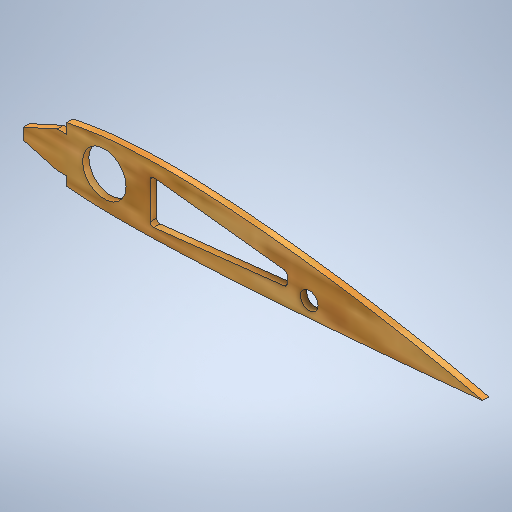
# Autodesk Inventor part: 2414 basic aerofoil
Saved by Autodesk Inventor 2025.1 (Build 291241000, 241)
## iProperties
Created: 2024-11-04
Part Number: 2414 basic aerofoil
Material: Plywood, Finish
Document SubType Name: Modeling
Designer: johan
Density: 0.552 g/cm^3
Appearance: Plywood - New
Author: johan
Autodesk Inventor part; units mm, degrees
ref_plane "YZ Plane" through (0, 0, 0) normal (1, 0, 0) x (0, 1, 0)
ref_plane "XZ Plane" through (0, 0, 0) normal (0, 1, 0) x (-1, 0, 0)
ref_plane "XY Plane" through (0, 0, 0) normal (0, 0, 1) x (1, 0, 0)
sketch "Sketch2" plane through (0, 0, 0) normal (0, 0, 1) x (1, 0, 0)
  spline S0 degree 5 poles (319.6498, 0.0573) (319.6501, 0.0612) (319.6024, 0.0717) (319.3745, 0.1032) (319.3587, 0.1577) (318.7204, 0.2502) (318.4411, 0.3675) (317.6227, 0.5236) (316.9347, 0.7102) (315.9239, 0.9334) (314.8763, 1.1861) (313.6258, 1.4728) (312.2675, 1.7887) (310.7514, 2.1347) (309.1071, 2.5099) (307.3204, 2.9131) (305.4017, 3.3421) (303.3481, 3.7974) (301.1639, 4.2757) (298.8502, 4.7782) (296.4092, 5.301) (293.8432, 5.8446) (291.1548, 6.4061) (288.3466, 6.9857) (285.4207, 7.5803) (282.3807, 8.1894) (279.2284, 8.8107) (275.968, 9.4437) (272.6016, 10.0865) (269.1329, 10.7361) (265.5656, 11.3942) (261.9019, 12.0551) (258.1469, 12.7207) (254.3029, 13.3883) (250.3742, 14.0555) (246.3647, 14.7217) (242.2776, 15.3854) (238.118, 16.0441) (233.8887, 16.6979) (229.5952, 17.3434) (225.2402, 17.981) (220.8297, 18.6074) (216.3658, 19.2226) (211.8552, 19.8242) (207.3009, 20.4107) (202.7077, 20.9813) (198.0804, 21.5339) (193.4232, 22.0679) (188.7413, 22.58) (184.0389, 23.0713) (179.321, 23.5382) (174.592, 23.982) (169.8567, 24.3971) (165.1201, 24.7874) (160.3872, 25.1472) (155.6604, 25.4776) (150.948, 25.7772) (146.2454, 26.0449) (141.5744, 26.278) (136.9015, 26.4795) (132.2479, 26.6311) (127.6319, 26.7393) (123.054, 26.7999) (118.5202, 26.8147) (114.0397, 26.7815) (109.6094, 26.7031) (105.2517, 26.5723) (100.9331, 26.4088) (96.7495, 26.1663) (92.5147, 25.9483) (88.6376, 25.5343) (84.2302, 25.3974) (76.5297, 24.5259) (73.18, 23.8676) (69.3619, 23.413) (65.9721, 22.8018) (62.3454, 22.244) (59.4319, 21.514) (55.4307, 21.0148) (53.2464, 20.1084) (49.5889, 19.537) (47.2944, 18.6473) (44.3884, 17.909) (41.914, 17.071) (39.4431, 16.2394) (37.1538, 15.3738) (34.9769, 14.4941) (32.9455, 13.5944) (31.0501, 12.6807) (29.2961, 11.7542) (27.6837, 10.8151) (26.2149, 9.8673) (24.8895, 8.9103) (23.7099, 7.9467) (22.6751, 6.976) (21.7868, 6.0004) (21.0458, 5.0186) (20.4526, 4.032) (20.0117, 3.0392) (19.7221, 2.0438) (19.5893, 1.0479) (19.6118, 0.0538) (19.7865, -0.9258) (20.1138, -1.8742) (20.591, -2.7944) (21.2165, -3.6796) (21.9855, -4.5321) (22.8956, -5.3514) (23.9453, -6.1385) (25.1332, -6.8944) (26.4582, -7.6188) (27.9184, -8.3123) (29.5136, -8.9751) (31.2409, -9.6071) (33.0997, -10.2067) (35.0892, -10.7758) (37.2002, -11.3131) (39.4562, -11.8174) (41.7927, -12.2939) (44.3651, -12.7275) (46.7744, -13.1584) (50.0005, -13.481) (52.1533, -13.8927) (55.9371, -14.1294) (58.2153, -14.4717) (61.732, -14.6854) (64.8012, -14.9153) (68.2287, -15.092) (71.6338, -15.2498) (75.1915, -15.3722) (78.8138, -15.4692) (82.5326, -15.5359) (86.3291, -15.5764) (90.2061, -15.5901) (94.1575, -15.5787) (98.1812, -15.5438) (102.2727, -15.4851) (106.4286, -15.4059) (110.6456, -15.3062) (114.9188, -15.1867) (119.2459, -15.0512) (123.6218, -14.8988) (128.0442, -14.7319) (132.5111, -14.552) (137.0141, -14.3592) (141.5621, -14.1606) (146.1675, -13.9403) (150.787, -13.7052) (155.434, -13.4523) (160.0951, -13.1857) (164.7676, -12.9046) (169.4465, -12.6129) (174.1261, -12.3082) (178.8033, -11.9955) (183.4722, -11.6727) (188.1294, -11.3426) (192.7696, -11.0072) (197.3886, -10.6641) (201.9818, -10.3188) (206.5448, -9.9678) (211.0728, -9.6157) (215.5623, -9.2611) (220.0069, -8.9047) (224.4048, -8.5497) (228.7492, -8.193) (233.0373, -7.8393) (237.2647, -7.4865) (241.4259, -7.1353) (245.5189, -6.7884) (249.5374, -6.4441) (253.4791, -6.104) (257.3389, -5.7683) (261.1136, -5.4376) (264.7987, -5.113) (268.3914, -4.7937) (271.8871, -4.4807) (275.2826, -4.1749) (278.5752, -3.8759) (281.7596, -3.585) (284.8354, -3.3021) (287.7962, -3.0278) (290.6419, -2.763) (293.3672, -2.5063) (295.9712, -2.2616) (298.4496, -2.0246) (300.8012, -1.801) (303.0222, -1.5859) (305.1122, -1.3849) (307.0656, -1.194) (308.8864, -1.0166) (310.5623, -0.8504) (312.1091, -0.6993) (313.4945, -0.5587) (314.7717, -0.4371) (315.8415, -0.3205) (316.8737, -0.2329) (317.5782, -0.1363) (318.4119, -0.0906) (318.7016, -0.0103) (319.3493, -0.0034) (319.3699, 0.0485) (319.6005, 0.0494) (319.6495, 0.0534) (319.6498, 0.0573) knots 0 0 0 0 0 0 1 2 3 4 5 6 7 8 9 10 11 12 13 14 15 16 17 18 19 20 21 22 23 24 25 26 27 28 29 30 31 32 33 34 35 36 37 38 39 40 41 42 43 44 45 46 47 48 49 50 51 52 53 54 55 56 57 58 59 60 61 62 63 64 65 66 67 68 69 70 71 72 73 74 75 76 77 78 79 80 81 82 83 84 85 86 87 88 89 90 91 92 93 94 95 96 97 98 99 100 101 102 103 104 105 106 107 108 109 110 111 112 113 114 115 116 117 118 119 120 121 122 123 124 125 126 127 128 129 130 131 132 133 134 135 136 137 138 139 140 141 142 143 144 145 146 147 148 149 150 151 152 153 154 155 156 157 158 159 160 161 162 163 164 165 166 167 168 169 170 171 172 173 174 175 176 177 178 179 180 181 182 183 184 185 186 187 188 189 190 191 192 193 194 195 196 197 198 199 199 199 199 199 199
  circle A0 centre (79.5137, 4.5678) radius 13.838
  line L0 (79.5137, 4.5678) -> (79.5137, -15.4763) construction
  line L1 (79.5137, 4.5678) -> (209.6498, 4.5678) construction
  line L2 (319.6498, 0.0573) -> (219.6498, 0.0573) construction
  line L3 (319.6498, 0.0573) -> (319.6498, 0.0574) construction
  line L4 (28.0058, 4.5054) -> (28.0058, -2.4946)
  line L5 (19.6272, 1.0326) -> (319.6498, 0.0573) construction
  line L6 (49.7105, 14.4213) -> (55.6078, 14.4213)
  line L7 (49.7104, -8.4914) -> (55.6078, -8.4914)
  line L8 (28.0058, 4.5054) -> (49.7105, 14.4213)
  line L9 (28.0058, -2.4946) -> (49.7104, -8.4914)
  line L10 (55.6078, 14.4213) -> (55.6078, 20.8729)
  line L11 (55.6078, -8.4914) -> (55.6078, -14.1513)
  line L12 (108.6496, 16.3299) -> (108.6496, -7.1942)
  line L13 (110.8735, -9.1817) -> (193.8736, 0.1678)
  line L14 (195.6498, 2.1552) -> (195.6498, 6.9805)
  line L15 (193.8736, 8.9679) -> (110.8735, 18.3173)
  arc A1 (110.8735, 18.3173) -> (108.6496, 16.3299) centre (110.6496, 16.3299) ccw
  arc A2 (108.6496, -7.1942) -> (110.8735, -9.1817) centre (110.6496, -7.1942) ccw
  arc A3 (193.8736, 0.1678) -> (195.6498, 2.1552) centre (193.6498, 2.1552) ccw
  arc A4 (195.6498, 6.9805) -> (193.8736, 8.9679) centre (193.6498, 6.9805) ccw
  circle A5 centre (209.6498, 0.0573) radius 5.661
  line L16 (319.6498, 0.0573) -> (319.6501, 0.0612) construction
  line L17 (319.6501, 0.0612) -> (319.6024, 0.0717) construction
  line L18 (319.6024, 0.0717) -> (319.3745, 0.1032) construction
  line L19 (319.3745, 0.1032) -> (319.3587, 0.1577) construction
  line L20 (319.3587, 0.1577) -> (318.7204, 0.2502) construction
  line L21 (318.7204, 0.2502) -> (318.4411, 0.3675) construction
  line L22 (318.4411, 0.3675) -> (317.6227, 0.5236) construction
  line L23 (317.6227, 0.5236) -> (316.9347, 0.7102) construction
  line L24 (316.9347, 0.7102) -> (315.9239, 0.9334) construction
  line L25 (315.9239, 0.9334) -> (314.8763, 1.1861) construction
  line L26 (314.8763, 1.1861) -> (313.6258, 1.4728) construction
  line L27 (313.6258, 1.4728) -> (312.2675, 1.7887) construction
  line L28 (312.2675, 1.7887) -> (310.7514, 2.1347) construction
  line L29 (310.7514, 2.1347) -> (309.1071, 2.5099) construction
  line L30 (309.1071, 2.5099) -> (307.3204, 2.9131) construction
  line L31 (307.3204, 2.9131) -> (305.4017, 3.3421) construction
  line L32 (305.4017, 3.3421) -> (303.3481, 3.7974) construction
  line L33 (303.3481, 3.7974) -> (301.1639, 4.2757) construction
  line L34 (301.1639, 4.2757) -> (298.8502, 4.7782) construction
  line L35 (298.8502, 4.7782) -> (296.4092, 5.301) construction
  line L36 (296.4092, 5.301) -> (293.8432, 5.8446) construction
  line L37 (293.8432, 5.8446) -> (291.1548, 6.4061) construction
  line L38 (291.1548, 6.4061) -> (288.3466, 6.9857) construction
  line L39 (288.3466, 6.9857) -> (285.4207, 7.5803) construction
  line L40 (285.4207, 7.5803) -> (282.3807, 8.1894) construction
  line L41 (282.3807, 8.1894) -> (279.2284, 8.8107) construction
  line L42 (279.2284, 8.8107) -> (275.968, 9.4437) construction
  line L43 (275.968, 9.4437) -> (272.6016, 10.0865) construction
  line L44 (272.6016, 10.0865) -> (269.1329, 10.7361) construction
  line L45 (269.1329, 10.7361) -> (265.5656, 11.3942) construction
  line L46 (265.5656, 11.3942) -> (261.9019, 12.0551) construction
  line L47 (261.9019, 12.0551) -> (258.1469, 12.7207) construction
  line L48 (258.1469, 12.7207) -> (254.3029, 13.3883) construction
  line L49 (254.3029, 13.3883) -> (250.3742, 14.0555) construction
  line L50 (250.3742, 14.0555) -> (246.3647, 14.7217) construction
  line L51 (246.3647, 14.7217) -> (242.2776, 15.3854) construction
  line L52 (242.2776, 15.3854) -> (238.118, 16.0441) construction
  line L53 (238.118, 16.0441) -> (233.8887, 16.6979) construction
  line L54 (233.8887, 16.6979) -> (229.5952, 17.3434) construction
  line L55 (229.5952, 17.3434) -> (225.2402, 17.981) construction
  line L56 (225.2402, 17.981) -> (220.8297, 18.6074) construction
  line L57 (220.8297, 18.6074) -> (216.3658, 19.2226) construction
  line L58 (216.3658, 19.2226) -> (211.8552, 19.8242) construction
  line L59 (211.8552, 19.8242) -> (207.3009, 20.4107) construction
  line L60 (207.3009, 20.4107) -> (202.7077, 20.9813) construction
  line L61 (202.7077, 20.9813) -> (198.0804, 21.5339) construction
  line L62 (198.0804, 21.5339) -> (193.4232, 22.0679) construction
  line L63 (193.4232, 22.0679) -> (188.7413, 22.58) construction
  line L64 (188.7413, 22.58) -> (184.0389, 23.0713) construction
  line L65 (184.0389, 23.0713) -> (179.321, 23.5382) construction
  line L66 (179.321, 23.5382) -> (174.592, 23.982) construction
  line L67 (174.592, 23.982) -> (169.8567, 24.3971) construction
  line L68 (169.8567, 24.3971) -> (165.1201, 24.7874) construction
  line L69 (165.1201, 24.7874) -> (160.3872, 25.1472) construction
  line L70 (160.3872, 25.1472) -> (155.6604, 25.4776) construction
  line L71 (155.6604, 25.4776) -> (150.948, 25.7772) construction
  line L72 (150.948, 25.7772) -> (146.2454, 26.0449) construction
  line L73 (146.2454, 26.0449) -> (141.5744, 26.278) construction
  line L74 (141.5744, 26.278) -> (136.9015, 26.4795) construction
  line L75 (136.9015, 26.4795) -> (132.2479, 26.6311) construction
  line L76 (132.2479, 26.6311) -> (127.6319, 26.7393) construction
  line L77 (127.6319, 26.7393) -> (123.054, 26.7999) construction
  line L78 (123.054, 26.7999) -> (118.5202, 26.8147) construction
  line L79 (118.5202, 26.8147) -> (114.0397, 26.7815) construction
  line L80 (114.0397, 26.7815) -> (109.6094, 26.7031) construction
  line L81 (109.6094, 26.7031) -> (105.2517, 26.5723) construction
  line L82 (105.2517, 26.5723) -> (100.9331, 26.4088) construction
  line L83 (100.9331, 26.4088) -> (96.7495, 26.1663) construction
  line L84 (96.7495, 26.1663) -> (92.5147, 25.9483) construction
  line L85 (92.5147, 25.9483) -> (88.6376, 25.5343) construction
  line L86 (88.6376, 25.5343) -> (84.2302, 25.3974) construction
  line L87 (84.2302, 25.3974) -> (76.5297, 24.5259) construction
  line L88 (76.5297, 24.5259) -> (73.18, 23.8676) construction
  line L89 (73.18, 23.8676) -> (69.3619, 23.413) construction
  line L90 (69.3619, 23.413) -> (65.9721, 22.8018) construction
  line L91 (65.9721, 22.8018) -> (62.3454, 22.244) construction
  line L92 (62.3454, 22.244) -> (59.4319, 21.514) construction
  line L93 (59.4319, 21.514) -> (55.4307, 21.0148) construction
  line L94 (55.4307, 21.0148) -> (53.2464, 20.1084) construction
  line L95 (53.2464, 20.1084) -> (49.5889, 19.537) construction
  line L96 (49.5889, 19.537) -> (47.2944, 18.6473) construction
  line L97 (47.2944, 18.6473) -> (44.3884, 17.909) construction
  line L98 (44.3884, 17.909) -> (41.914, 17.071) construction
  line L99 (41.914, 17.071) -> (39.4431, 16.2394) construction
  line L100 (39.4431, 16.2394) -> (37.1538, 15.3738) construction
  line L101 (37.1538, 15.3738) -> (34.9769, 14.4941) construction
  line L102 (34.9769, 14.4941) -> (32.9455, 13.5944) construction
  line L103 (32.9455, 13.5944) -> (31.0501, 12.6807) construction
  line L104 (31.0501, 12.6807) -> (29.2961, 11.7542) construction
  line L105 (29.2961, 11.7542) -> (27.6837, 10.8151) construction
  line L106 (27.6837, 10.8151) -> (26.2149, 9.8673) construction
  line L107 (26.2149, 9.8673) -> (24.8895, 8.9103) construction
  line L108 (24.8895, 8.9103) -> (23.7099, 7.9467) construction
  line L109 (23.7099, 7.9467) -> (22.6751, 6.976) construction
  line L110 (22.6751, 6.976) -> (21.7868, 6.0004) construction
  line L111 (21.7868, 6.0004) -> (21.0458, 5.0186) construction
  line L112 (21.0458, 5.0186) -> (20.4526, 4.032) construction
  line L113 (20.4526, 4.032) -> (20.0117, 3.0392) construction
  line L114 (20.0117, 3.0392) -> (19.7221, 2.0438) construction
  line L115 (19.7221, 2.0438) -> (19.5893, 1.0479) construction
  line L116 (19.5893, 1.0479) -> (19.6118, 0.0538) construction
  line L117 (19.6118, 0.0538) -> (19.7865, -0.9258) construction
  line L118 (19.7865, -0.9258) -> (20.1138, -1.8742) construction
  line L119 (20.1138, -1.8742) -> (20.591, -2.7944) construction
  line L120 (20.591, -2.7944) -> (21.2165, -3.6796) construction
  line L121 (21.2165, -3.6796) -> (21.9855, -4.5321) construction
  line L122 (21.9855, -4.5321) -> (22.8956, -5.3514) construction
  line L123 (22.8956, -5.3514) -> (23.9453, -6.1385) construction
  line L124 (23.9453, -6.1385) -> (25.1332, -6.8944) construction
  line L125 (25.1332, -6.8944) -> (26.4582, -7.6188) construction
  line L126 (26.4582, -7.6188) -> (27.9184, -8.3123) construction
  line L127 (27.9184, -8.3123) -> (29.5136, -8.9751) construction
  line L128 (29.5136, -8.9751) -> (31.2409, -9.6071) construction
  line L129 (31.2409, -9.6071) -> (33.0997, -10.2067) construction
  line L130 (33.0997, -10.2067) -> (35.0892, -10.7758) construction
  line L131 (35.0892, -10.7758) -> (37.2002, -11.3131) construction
  line L132 (37.2002, -11.3131) -> (39.4562, -11.8174) construction
  line L133 (39.4562, -11.8174) -> (41.7927, -12.2939) construction
  line L134 (41.7927, -12.2939) -> (44.3651, -12.7275) construction
  line L135 (44.3651, -12.7275) -> (46.7744, -13.1584) construction
  line L136 (46.7744, -13.1584) -> (50.0005, -13.481) construction
  line L137 (50.0005, -13.481) -> (52.1533, -13.8927) construction
  line L138 (52.1533, -13.8927) -> (55.9371, -14.1294) construction
  line L139 (55.9371, -14.1294) -> (58.2153, -14.4717) construction
  line L140 (58.2153, -14.4717) -> (61.732, -14.6854) construction
  line L141 (61.732, -14.6854) -> (64.8012, -14.9153) construction
  line L142 (64.8012, -14.9153) -> (68.2287, -15.092) construction
  line L143 (68.2287, -15.092) -> (71.6338, -15.2498) construction
  line L144 (71.6338, -15.2498) -> (75.1915, -15.3722) construction
  line L145 (75.1915, -15.3722) -> (78.8138, -15.4692) construction
  line L146 (78.8138, -15.4692) -> (82.5326, -15.5359) construction
  line L147 (82.5326, -15.5359) -> (86.3291, -15.5764) construction
  line L148 (86.3291, -15.5764) -> (90.2061, -15.5901) construction
  line L149 (90.2061, -15.5901) -> (94.1575, -15.5787) construction
  line L150 (94.1575, -15.5787) -> (98.1812, -15.5438) construction
  line L151 (98.1812, -15.5438) -> (102.2727, -15.4851) construction
  line L152 (102.2727, -15.4851) -> (106.4286, -15.4059) construction
  line L153 (106.4286, -15.4059) -> (110.6456, -15.3062) construction
  line L154 (110.6456, -15.3062) -> (114.9188, -15.1867) construction
  line L155 (114.9188, -15.1867) -> (119.2459, -15.0512) construction
  line L156 (119.2459, -15.0512) -> (123.6218, -14.8988) construction
  line L157 (123.6218, -14.8988) -> (128.0442, -14.7319) construction
  line L158 (128.0442, -14.7319) -> (132.5111, -14.552) construction
  line L159 (132.5111, -14.552) -> (137.0141, -14.3592) construction
  line L160 (137.0141, -14.3592) -> (141.5621, -14.1606) construction
  line L161 (141.5621, -14.1606) -> (146.1675, -13.9403) construction
  line L162 (146.1675, -13.9403) -> (150.787, -13.7052) construction
  line L163 (150.787, -13.7052) -> (155.434, -13.4523) construction
  line L164 (155.434, -13.4523) -> (160.0951, -13.1857) construction
  line L165 (160.0951, -13.1857) -> (164.7676, -12.9046) construction
  line L166 (164.7676, -12.9046) -> (169.4465, -12.6129) construction
  line L167 (169.4465, -12.6129) -> (174.1261, -12.3082) construction
  line L168 (174.1261, -12.3082) -> (178.8033, -11.9955) construction
  line L169 (178.8033, -11.9955) -> (183.4722, -11.6727) construction
  line L170 (183.4722, -11.6727) -> (188.1294, -11.3426) construction
  line L171 (188.1294, -11.3426) -> (192.7696, -11.0072) construction
  line L172 (192.7696, -11.0072) -> (197.3886, -10.6641) construction
  line L173 (197.3886, -10.6641) -> (201.9818, -10.3188) construction
  line L174 (201.9818, -10.3188) -> (206.5448, -9.9678) construction
  line L175 (206.5448, -9.9678) -> (211.0728, -9.6157) construction
  line L176 (211.0728, -9.6157) -> (215.5623, -9.2611) construction
  line L177 (215.5623, -9.2611) -> (220.0069, -8.9047) construction
  line L178 (220.0069, -8.9047) -> (224.4048, -8.5497) construction
  line L179 (224.4048, -8.5497) -> (228.7492, -8.193) construction
  line L180 (228.7492, -8.193) -> (233.0373, -7.8393) construction
  line L181 (233.0373, -7.8393) -> (237.2647, -7.4865) construction
  line L182 (237.2647, -7.4865) -> (241.4259, -7.1353) construction
  line L183 (241.4259, -7.1353) -> (245.5189, -6.7884) construction
  line L184 (245.5189, -6.7884) -> (249.5374, -6.4441) construction
  line L185 (249.5374, -6.4441) -> (253.4791, -6.104) construction
  line L186 (253.4791, -6.104) -> (257.3389, -5.7683) construction
  line L187 (257.3389, -5.7683) -> (261.1136, -5.4376) construction
  line L188 (261.1136, -5.4376) -> (264.7987, -5.113) construction
  line L189 (264.7987, -5.113) -> (268.3914, -4.7937) construction
  line L190 (268.3914, -4.7937) -> (271.8871, -4.4807) construction
  line L191 (271.8871, -4.4807) -> (275.2826, -4.1749) construction
  line L192 (275.2826, -4.1749) -> (278.5752, -3.8759) construction
  line L193 (278.5752, -3.8759) -> (281.7596, -3.585) construction
  line L194 (281.7596, -3.585) -> (284.8354, -3.3021) construction
  line L195 (284.8354, -3.3021) -> (287.7962, -3.0278) construction
  line L196 (287.7962, -3.0278) -> (290.6419, -2.763) construction
  line L197 (290.6419, -2.763) -> (293.3672, -2.5063) construction
  line L198 (293.3672, -2.5063) -> (295.9712, -2.2616) construction
  line L199 (295.9712, -2.2616) -> (298.4496, -2.0246) construction
  line L200 (298.4496, -2.0246) -> (300.8012, -1.801) construction
  line L201 (300.8012, -1.801) -> (303.0222, -1.5859) construction
  line L202 (303.0222, -1.5859) -> (305.1122, -1.3849) construction
  line L203 (305.1122, -1.3849) -> (307.0656, -1.194) construction
  line L204 (307.0656, -1.194) -> (308.8864, -1.0166) construction
  line L205 (308.8864, -1.0166) -> (310.5623, -0.8504) construction
  line L206 (310.5623, -0.8504) -> (312.1091, -0.6993) construction
  line L207 (312.1091, -0.6993) -> (313.4945, -0.5587) construction
  line L208 (313.4945, -0.5587) -> (314.7717, -0.4371) construction
  line L209 (314.7717, -0.4371) -> (315.8415, -0.3205) construction
  line L210 (315.8415, -0.3205) -> (316.8737, -0.2329) construction
  line L211 (316.8737, -0.2329) -> (317.5782, -0.1363) construction
  line L212 (317.5782, -0.1363) -> (318.4119, -0.0906) construction
  line L213 (318.4119, -0.0906) -> (318.7016, -0.0103) construction
  line L214 (318.7016, -0.0103) -> (319.3493, -0.0034) construction
  line L215 (319.3493, -0.0034) -> (319.3699, 0.0485) construction
  line L216 (319.3699, 0.0485) -> (319.6005, 0.0494) construction
  line L217 (319.6005, 0.0494) -> (319.6495, 0.0534) construction
  line L218 (319.6495, 0.0534) -> (319.6498, 0.0573) construction
  point P0 (0, 0)
  point P1 (319.5771, 0.0748)
  point P2 (319.3573, 0.1272)
  point P3 (318.9916, 0.2136)
  point P4 (318.4804, 0.3362)
  point P5 (317.8238, 0.4909)
  point P6 (317.0222, 0.6802)
  point P7 (316.0769, 0.9024)
  point P8 (314.9885, 1.1569)
  point P9 (313.7582, 1.443)
  point P10 (312.3866, 1.7598)
  point P11 (310.8752, 2.1063)
  point P12 (309.2258, 2.4819)
  point P13 (307.4393, 2.8854)
  point P14 (305.5178, 3.3153)
  point P15 (303.4628, 3.7707)
  point P16 (301.2764, 4.2501)
  point P17 (298.9607, 4.7526)
  point P18 (296.5175, 5.2764)
  point P19 (293.9492, 5.8203)
  point P20 (291.2585, 6.3828)
  point P21 (288.4478, 6.9627)
  point P22 (285.5195, 7.5582)
  point P23 (282.4766, 8.1678)
  point P24 (279.3218, 8.79)
  point P25 (276.0584, 9.4236)
  point P26 (272.6891, 10.0668)
  point P27 (269.2175, 10.7178)
  point P28 (265.6469, 11.3757)
  point P29 (261.9803, 12.0381)
  point P30 (258.2219, 12.7041)
  point P31 (254.3747, 13.3722)
  point P32 (250.4426, 14.0403)
  point P33 (246.4295, 14.7072)
  point P34 (242.339, 15.3714)
  point P35 (238.1756, 16.0311)
  point P36 (233.9428, 16.6851)
  point P37 (229.6454, 17.3316)
  point P38 (225.2869, 17.9694)
  point P39 (220.8723, 18.5967)
  point P40 (216.4049, 19.2123)
  point P41 (211.8901, 19.8144)
  point P42 (207.332, 20.4015)
  point P43 (202.7347, 20.9724)
  point P44 (198.1034, 21.5256)
  point P45 (193.4423, 22.0596)
  point P46 (188.7563, 22.5726)
  point P47 (184.0499, 23.0637)
  point P48 (179.3279, 23.5314)
  point P49 (174.5948, 23.9745)
  point P50 (169.8554, 24.3909)
  point P51 (165.1148, 24.7803)
  point P52 (160.3775, 25.1406)
  point P53 (155.6479, 25.4709)
  point P54 (150.9316, 25.7703)
  point P55 (146.233, 26.0373)
  point P56 (141.557, 26.2707)
  point P57 (136.8821, 26.4681)
  point P58 (132.2209, 26.6211)
  point P59 (127.5964, 26.7282)
  point P60 (123.0133, 26.7888)
  point P61 (118.4761, 26.8026)
  point P62 (113.9902, 26.7693)
  point P63 (109.5601, 26.6886)
  point P64 (105.191, 26.5611)
  point P65 (100.8865, 26.3866)
  point P66 (96.6524, 26.1647)
  point P67 (92.4927, 25.8975)
  point P68 (88.412, 25.5858)
  point P69 (84.409, 25.3061)
  point P70 (80.8803, 24.9766)
  point P71 (76.6761, 24.4558)
  point P72 (72.9631, 23.8932)
  point P73 (69.3402, 23.3612)
  point P74 (65.8208, 22.7938)
  point P75 (62.4086, 22.1884)
  point P76 (59.1071, 21.5462)
  point P77 (52.8493, 20.1606)
  point P78 (49.7105, 19.4213)
  point P79 (47.0737, 18.6508)
  point P80 (44.3741, 17.8542)
  point P81 (41.8033, 17.0323)
  point P82 (39.3638, 16.1875)
  point P83 (37.0582, 15.3214)
  point P84 (34.8883, 14.4364)
  point P85 (32.8567, 13.534)
  point P86 (30.9649, 12.6166)
  point P87 (29.2144, 11.686)
  point P88 (27.607, 10.7437)
  point P89 (26.1442, 9.7921)
  point P90 (24.8269, 8.8324)
  point P91 (23.6566, 7.8664)
  point P92 (22.6337, 6.8952)
  point P93 (21.7592, 5.9208)
  point P94 (21.0335, 4.944)
  point P95 (20.4573, 3.966)
  point P96 (20.031, 2.9874)
  point P97 (19.7541, 2.0097)
  point P98 (19.6496, 0.0598)
  point P99 (19.8207, -0.9032)
  point P100 (20.1378, -1.8356)
  point P101 (20.6004, -2.7401)
  point P102 (21.2081, -3.6158)
  point P103 (21.9599, -4.4627)
  point P104 (22.8545, -5.2806)
  point P105 (23.891, -6.069)
  point P106 (25.0682, -6.8277)
  point P107 (26.3845, -7.5561)
  point P108 (27.8383, -8.2539)
  point P109 (29.4283, -8.9211)
  point P110 (31.1522, -9.5571)
  point P111 (33.0086, -10.1613)
  point P112 (34.9949, -10.734)
  point P113 (37.1093, -11.2746)
  point P114 (39.3497, -11.7828)
  point P115 (41.7134, -12.2586)
  point P116 (44.1979, -12.702)
  point P117 (46.8014, -13.1127)
  point P118 (49.7104, -13.4914)
  point P119 (52.3532, -13.8357)
  point P120 (58.3469, -14.4294)
  point P121 (61.5023, -14.678)
  point P122 (64.7591, -14.8953)
  point P123 (68.1149, -15.0813)
  point P124 (71.5661, -15.237)
  point P125 (75.1094, -15.3627)
  point P126 (78.7418, -15.4596)
  point P127 (82.46, -15.528)
  point P128 (86.2607, -15.5691)
  point P129 (90.14, -15.5838)
  point P130 (94.0946, -15.5733)
  point P131 (98.1212, -15.5388)
  point P132 (102.2159, -15.4812)
  point P133 (106.3751, -15.4023)
  point P134 (110.5952, -15.303)
  point P135 (114.872, -15.1845)
  point P136 (119.2022, -15.0489)
  point P137 (123.5813, -14.8971)
  point P138 (128.006, -14.7306)
  point P139 (132.4718, -14.5509)
  point P140 (136.9748, -14.3598)
  point P141 (141.5285, -14.1576)
  point P142 (146.1365, -13.9383)
  point P143 (150.7679, -13.7022)
  point P144 (155.4191, -13.4499)
  point P145 (160.0853, -13.1829)
  point P146 (164.7617, -12.9024)
  point P147 (169.4444, -12.6099)
  point P148 (174.1283, -12.306)
  point P149 (178.8092, -11.9925)
  point P150 (183.4823, -11.67)
  point P151 (188.1434, -11.34)
  point P152 (192.7877, -11.0037)
  point P153 (197.4107, -10.6614)
  point P154 (202.0079, -10.3149)
  point P155 (206.5747, -9.9645)
  point P156 (211.1069, -9.6117)
  point P157 (215.5999, -9.2568)
  point P158 (220.0489, -8.9007)
  point P159 (224.4503, -8.5446)
  point P160 (228.7987, -8.1885)
  point P161 (233.0906, -7.8339)
  point P162 (237.3214, -7.4808)
  point P163 (241.4866, -7.1298)
  point P164 (245.5828, -6.7821)
  point P165 (249.6052, -6.4377)
  point P166 (253.5502, -6.0972)
  point P167 (257.4136, -5.7612)
  point P168 (261.1915, -5.4303)
  point P169 (264.88, -5.1051)
  point P170 (268.4758, -4.7856)
  point P171 (271.9747, -4.4724)
  point P172 (275.3734, -4.1661)
  point P173 (278.6686, -3.867)
  point P174 (281.8564, -3.5757)
  point P175 (284.9344, -3.2925)
  point P176 (287.8984, -3.018)
  point P177 (290.7463, -2.7525)
  point P178 (293.4745, -2.4963)
  point P179 (296.0806, -2.2503)
  point P180 (298.5616, -2.0142)
  point P181 (300.9151, -1.7892)
  point P182 (303.1387, -1.575)
  point P183 (305.23, -1.3728)
  point P184 (307.1866, -1.1823)
  point P185 (309.007, -1.0041)
  point P186 (310.6885, -0.8385)
  point P187 (312.2302, -0.6861)
  point P188 (313.6297, -0.5471)
  point P189 (314.8861, -0.4221)
  point P190 (315.9976, -0.3107)
  point P191 (316.9636, -0.214)
  point P192 (317.7826, -0.1311)
  point P193 (318.4538, -0.0643)
  point P194 (318.9765, -0.0102)
  point P195 (319.3503, 0.027)
  point P196 (319.5743, 0.0497)
  point P197 (28.0058, 1.0054)
  point P198 (108.6496, 18.5678)
  point P199 (108.6496, -9.4322)
  dimension "d2" = 300.0001
  dimension "d19" = 110
  dimension "d22" = 100
  dimension "d23" = 7
  dimension "d24" = 5
  dimension "d25" = 5
  dimension "d30" = 28
  dimension "d31" = 8.4
  dimension "d33" = 14
  dimension "d34" = 2
  dimension "d37" = 27.676
  dimension "d40" = 11.322
  dimension "d42" = 59.8865
  constraints: 32 end point, 11 point on line, 8 point on circle, 8 tangent, 6 centre point, 5 vertical, 3 equal radius, 3 midpoint, 2 horizontal, 1 horizontal alignment, 1 parallel, 1 perpendicular, 1 vertical alignment, 203 other
  measures "d2" distance of L2.start point (19.65, 0.06)
  measures "d19" horizontal distance of L2.start L1.end
  measures "d22" distance of L2.start L2.end
  measures "d23" distance of L4.start L4.end
  measures "d24" distance from line of point (49.71, 19.421) L6
  measures "d25" distance from line of point (49.71, -13.491) L7
  measures "d30" distance of point (108.65, 18.568) point (108.65, -9.432)
  measures "d31" distance of point (195.65, 0.368) point (195.65, 8.768)
  measures "d33" distance from line of L1.end L14
  measures "d34" radius of A1
  measures "d37" diameter of A0
  measures "d40" diameter of A5
  measures "d42" horizontal distance of L5.start L0.start
extrude "Extrusion6" add sketch "Sketch2" along normal blind 4 contours S0 L11 L7 L9 L4 L8 L6 L10 picked at (250.5476, 2.1053)
body "Solid6"
